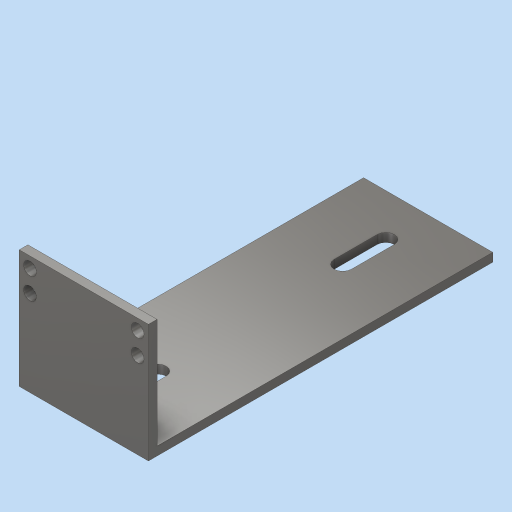
# Autodesk Inventor part: Spoj stolu a kolejnice
Saved by Autodesk Inventor 2024 (Build 280153000, 153)
## iProperties
Created: 2021-04-14
Part Number: Spoj stolu a kolejnice
Material: Steel, Cast
Document SubType Name: Modeling
Designer: Karbosch
Density: 7.85 g/cm^3
Appearance: Semi-Polished
Mass: 380.768 g
Surface Area: 272.434 cm^2
Volume: 48.5055 cm^3
Author: Karbosch
Autodesk Inventor part; units mm, degrees
ref_plane "YZ Plane" through (0, 0, 0) normal (1, 0, 0) x (0, 1, 0)
ref_plane "XZ Plane" through (0, 0, 0) normal (0, 1, 0) x (-1, 0, 0)
sketch "Sketch21" plane through (0, 0, 0) normal (0, 1, 0) x (-1, 0, 0)
  line L0 (4, -34.3) -> (4, -14.3)
  line L1 (-4, -14.3) -> (-4, -34.3)
  arc A0 (-4, -34.3) -> (4, -34.3) centre (0, -34.3) ccw
  arc A1 (4, -14.3) -> (-4, -14.3) centre (0, -14.3) ccw
  arc A2 (-4, -140.3) -> (4, -140.3) centre (0, -140.3) ccw
  line L2 (-4, -140.3) -> (-4, -120.3)
  arc A3 (4, -120.3) -> (-4, -120.3) centre (0, -120.3) ccw
  line L3 (4, -140.3) -> (4, -120.3)
  line L4 (0, -14.3) -> (59.397, -14.3) construction
  line L5 (0, -14.3) -> (69.2965, -14.3) construction
  line L6 (-30, 0) -> (30, 0)
  line L7 (30, 0) -> (30, -160)
  line L8 (30, -160) -> (-30, -160)
  line L9 (-30, -160) -> (-30, 0)
  point P0 (0, 0)
  dimension "d114" = 8
  dimension "d115" = 20
  dimension "d116" = 8
  dimension "d118" = 20
  dimension "d146" = 60
  constraints: 20 end point, 8 point on circle, 4 centre point, 3 horizontal, 3 vertical, 2 parallel, 1 perpendicular
  measures "d114" distance of L1.end L0.start
  measures "d115" distance of L0.start L0.end
  measures "d116" distance of L0.end L1.start
  measures "d118" distance of L2.start L2.end
  measures "d146" distance of L7.end L8.end
ref_plane "Work Plane7" through (-35, 0, 0) normal (0, 0, 1) x (1, 0, 0)
sketch "Sketch22" plane through (-35, 0, 0) normal (0, 0, 1) x (1, 0, 0)
  circle A0 centre (10, 40) radius 3
  circle A1 centre (60, 40) radius 3
  line L0 (65, 55) -> (5, 55)
  line L1 (5, 55) -> (5, 0)
  line L2 (5, 0) -> (65, 0)
  line L3 (65, 0) -> (65, 55)
  circle A2 centre (60, 50) radius 3
  circle A3 centre (10, 50) radius 3
  point P0 (35, 0)
  point P1 (0, 0)
  dimension "d121" = 6
  dimension "d122" = 6
  dimension "d151" = 6
  dimension "d152" = 6
  constraints: 8 end point, 4 centre point, 2 parallel, 1 horizontal, 1 perpendicular
  measures "d121" diameter of A0
  measures "d122" diameter of A1
  measures "d151" diameter of A2
  measures "d152" diameter of A3
extrude "Extrusion13" add sketch "Sketch21" along normal blind 4
extrude "Extrusion15" add sketch "Sketch22" against normal blind 4
sketch "Sketch24" plane through (0, 4, 0) normal (0, 1, 0) x (1, 0, 0)
  line L0 (4, 120.3) -> (4, 140.3) projected
  line L1 (4, 130.3) -> (-4, 130.3)
  line L2 (-4, 140.3) -> (-4, 120.3) projected
  line L3 (4, 14.3) -> (4, 34.3) projected
  line L4 (4, 24.3) -> (-4, 24.3)
  line L5 (-4, 34.3) -> (-4, 14.3) projected
  circle A0 centre (0, 130.3) radius 4
  circle A1 centre (0, 24.3) radius 4
  point P0 (0, 0)
  constraints: 6 midpoint, 4 end point, 1 centre point, 1 horizontal alignment, 1 tangent, 2 other
body "Solid3"
